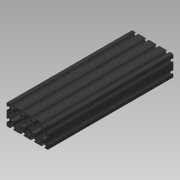
# Autodesk Inventor part: 2040
Saved by Autodesk Inventor 2013 (Build 170138000, 138)
## iProperties
Company: 80/20 Inc.
Created: 2013-09-06
Part Number: 2040
Material: Generic
Document SubType Name: Modeling
Density: 1 g/cm^3
Catalog Web Link: 8020.net
Vendor: 80/20 Inc.
Engineer: Ross Bowman
Author: Ross Bowman
Keywords: T-Slot, Extrusion, 80/20, 8020, Quick Frame, HT
Autodesk Inventor part; units mm, degrees
ref_plane "YZ Plane" through (0, 0, 0) normal (1, 0, 0) x (0, 1, 0)
ref_plane "XZ Plane" through (0, 0, 0) normal (0, 1, 0) x (-1, 0, 0)
ref_plane "XY Plane" through (0, 0, 0) normal (0, 0, 1) x (1, 0, 0)
sketch "Sketch1" plane through (0, 0, 0) normal (0, 0, 1) x (1, 0, 0)
  circle A0 centre (-12.7, 12.7) radius 2.6035
  circle A1 centre (-12.7, -12.7) radius 2.6035
  circle A2 centre (-38.1, 12.7) radius 2.6035
  circle A3 centre (-38.1, -12.7) radius 2.6035
  circle A4 centre (12.7, 12.7) radius 2.6035
  circle A5 centre (12.7, -12.7) radius 2.6035
  circle A6 centre (38.1, 12.7) radius 2.6035
  circle A7 centre (38.1, -12.7) radius 2.6035
  line L0 (-7.2742, 8.8373) -> (-2.0654, 3.6286)
  arc A8 (-2.0654, 3.6286) -> (2.0654, 3.6286) centre (0, 5.6941) ccw
  line L1 (2.0654, 3.6286) -> (7.2742, 8.8373)
  arc A9 (7.2742, 8.8373) -> (8.2042, 11.0824) centre (5.0292, 11.0824) ccw
  line L2 (8.2042, 11.0824) -> (8.2042, 14.3186)
  arc A10 (8.2042, 14.3186) -> (7.2743, 16.5636) centre (5.0292, 14.3186) ccw
  line L3 (7.2743, 16.5636) -> (2.0655, 21.7725)
  arc A11 (2.0655, 21.7725) -> (-2.0655, 21.7725) centre (0, 19.7071) ccw
  line L4 (-2.0655, 21.7725) -> (-7.2743, 16.5636)
  arc A12 (-7.2743, 16.5636) -> (-8.2042, 14.3186) centre (-5.0292, 14.3186) ccw
  line L5 (-8.2042, 14.3186) -> (-8.2042, 11.0824)
  arc A13 (-8.2042, 11.0824) -> (-7.2742, 8.8373) centre (-5.0292, 11.0824) ccw
  line L6 (-7.2743, -16.5636) -> (-2.0655, -21.7725)
  arc A14 (-2.0655, -21.7725) -> (2.0655, -21.7725) centre (0, -19.7071) ccw
  line L7 (2.0655, -21.7725) -> (7.2743, -16.5636)
  arc A15 (7.2743, -16.5636) -> (8.2042, -14.3186) centre (5.0292, -14.3186) ccw
  line L8 (8.2042, -14.3186) -> (8.2042, -11.0824)
  arc A16 (8.2042, -11.0824) -> (7.2742, -8.8373) centre (5.0292, -11.0824) ccw
  line L9 (7.2742, -8.8373) -> (2.0654, -3.6286)
  arc A17 (2.0654, -3.6286) -> (-2.0654, -3.6286) centre (0, -5.6941) ccw
  line L10 (-2.0654, -3.6286) -> (-7.2742, -8.8373)
  arc A18 (-7.2742, -8.8373) -> (-8.2042, -11.0824) centre (-5.0292, -11.0824) ccw
  line L11 (-8.2042, -11.0824) -> (-8.2042, -14.3186)
  arc A19 (-8.2042, -14.3186) -> (-7.2743, -16.5636) centre (-5.0292, -14.3186) ccw
  line L12 (-17.1958, 10.414) -> (-17.1958, 14.7184)
  arc A20 (-17.1958, 14.7184) -> (-17.843, 16.2809) centre (-19.4056, 14.7184) ccw
  line L13 (-17.843, 16.2809) -> (-23.3345, 21.7725)
  arc A21 (-23.3345, 21.7725) -> (-27.4655, 21.7725) centre (-25.4, 19.7071) ccw
  line L14 (-27.4655, 21.7725) -> (-32.957, 16.2809)
  arc A22 (-32.957, 16.2809) -> (-33.6042, 14.7184) centre (-31.3944, 14.7184) ccw
  line L15 (-33.6042, 14.7184) -> (-33.6042, 10.414)
  arc A23 (-35.814, 8.2042) -> (-33.6042, 10.414) centre (-35.814, 10.414) ccw
  line L16 (-35.814, 8.2042) -> (-40.1184, 8.2042)
  arc A24 (-40.1184, 8.2042) -> (-41.6809, 7.557) centre (-40.1184, 5.9944) ccw
  line L17 (-41.6809, 7.557) -> (-47.1725, 2.0655)
  arc A25 (-47.1725, 2.0655) -> (-47.1725, -2.0655) centre (-45.1071, 0) ccw
  line L18 (-47.1725, -2.0655) -> (-41.6809, -7.557)
  arc A26 (-41.6809, -7.557) -> (-40.1184, -8.2042) centre (-40.1184, -5.9944) ccw
  line L19 (-40.1184, -8.2042) -> (-35.814, -8.2042)
  arc A27 (-33.6042, -10.414) -> (-35.814, -8.2042) centre (-35.814, -10.414) ccw
  line L20 (-33.6042, -10.414) -> (-33.6042, -14.7184)
  arc A28 (-33.6042, -14.7184) -> (-32.957, -16.2809) centre (-31.3944, -14.7184) ccw
  line L21 (-32.957, -16.2809) -> (-27.4655, -21.7725)
  arc A29 (-27.4655, -21.7725) -> (-23.3345, -21.7725) centre (-25.4, -19.7071) ccw
  line L22 (-23.3345, -21.7725) -> (-17.843, -16.2809)
  arc A30 (-17.843, -16.2809) -> (-17.1958, -14.7184) centre (-19.4056, -14.7184) ccw
  line L23 (-17.1958, -14.7184) -> (-17.1958, -10.414)
  arc A31 (-14.986, -8.2042) -> (-17.1958, -10.414) centre (-14.986, -10.414) ccw
  line L24 (-14.986, -8.2042) -> (-10.6816, -8.2042)
  arc A32 (-10.6816, -8.2042) -> (-9.1191, -7.557) centre (-10.6816, -5.9944) ccw
  line L25 (-9.1191, -7.557) -> (-3.6275, -2.0655)
  arc A33 (-3.6275, -2.0655) -> (-3.6275, 2.0655) centre (-5.6929, 0) ccw
  line L26 (-3.6275, 2.0655) -> (-9.1191, 7.557)
  arc A34 (-9.1191, 7.557) -> (-10.6816, 8.2042) centre (-10.6816, 5.9944) ccw
  line L27 (-10.6816, 8.2042) -> (-14.986, 8.2042)
  arc A35 (-17.1958, 10.414) -> (-14.986, 8.2042) centre (-14.986, 10.414) ccw
  line L28 (14.986, 8.2042) -> (10.6816, 8.2042)
  arc A36 (10.6816, 8.2042) -> (9.1191, 7.557) centre (10.6816, 5.9944) ccw
  line L29 (9.1191, 7.557) -> (3.6275, 2.0655)
  arc A37 (3.6275, 2.0655) -> (3.6275, -2.0655) centre (5.6929, 0) ccw
  line L30 (3.6275, -2.0655) -> (9.1191, -7.557)
  arc A38 (9.1191, -7.557) -> (10.6816, -8.2042) centre (10.6816, -5.9944) ccw
  line L31 (10.6816, -8.2042) -> (14.986, -8.2042)
  arc A39 (17.1958, -10.414) -> (14.986, -8.2042) centre (14.986, -10.414) ccw
  line L32 (17.1958, -10.414) -> (17.1958, -14.7184)
  arc A40 (17.1958, -14.7184) -> (17.843, -16.2809) centre (19.4056, -14.7184) ccw
  line L33 (17.843, -16.2809) -> (23.3345, -21.7725)
  arc A41 (23.3345, -21.7725) -> (27.4655, -21.7725) centre (25.4, -19.7071) ccw
  line L34 (27.4655, -21.7725) -> (32.957, -16.2809)
  line L35 (33.6042, -14.7184) -> (33.6042, -10.414)
  arc A42 (35.814, -8.2042) -> (33.6042, -10.414) centre (35.814, -10.414) ccw
  line L36 (35.814, -8.2042) -> (40.1184, -8.2042)
  arc A43 (40.1184, -8.2042) -> (41.6809, -7.557) centre (40.1184, -5.9944) ccw
  line L37 (41.6809, -7.557) -> (47.1725, -2.0655)
  arc A44 (47.1725, -2.0655) -> (47.1725, 2.0655) centre (45.1071, 0) ccw
  line L38 (47.1725, 2.0655) -> (41.6809, 7.557)
  arc A45 (41.6809, 7.557) -> (40.1184, 8.2042) centre (40.1184, 5.9944) ccw
  line L39 (40.1184, 8.2042) -> (35.814, 8.2042)
  arc A46 (33.6042, 10.414) -> (35.814, 8.2042) centre (35.814, 10.414) ccw
  line L40 (33.6042, 10.414) -> (33.6042, 14.7184)
  arc A47 (33.6042, 14.7184) -> (32.957, 16.2809) centre (31.3944, 14.7184) ccw
  line L41 (32.957, 16.2809) -> (27.4655, 21.7725)
  arc A48 (27.4655, 21.7725) -> (23.3345, 21.7725) centre (25.4, 19.7071) ccw
  line L42 (23.3345, 21.7725) -> (17.843, 16.2809)
  arc A49 (17.843, 16.2809) -> (17.1958, 14.7184) centre (19.4056, 14.7184) ccw
  line L43 (17.1958, 14.7184) -> (17.1958, 10.414)
  arc A50 (14.986, 8.2042) -> (17.1958, 10.414) centre (14.986, 10.414) ccw
  arc A51 (32.957, -16.2809) -> (33.6042, -14.7184) centre (31.3944, -14.7184) ccw
  line L44 (2.1336, 25.4) -> (-2.1336, 25.4)
  arc A52 (-3.1496, 25.4) -> (-2.1336, 25.4) centre (-2.6416, 25.4) ccw
  line L45 (-3.1496, 25.4) -> (-6.096, 25.4)
  arc A53 (-7.112, 25.4) -> (-6.096, 25.4) centre (-6.604, 25.4) ccw
  line L46 (-7.112, 25.4) -> (-8.3566, 25.4)
  arc A54 (-8.3566, 25.4) -> (-8.3566, 23.1902) centre (-8.357, 24.2951) ccw
  line L47 (-8.3566, 23.1902) -> (-6.2257, 23.1902)
  arc A55 (-5.5073, 21.4558) -> (-6.2257, 23.1902) centre (-6.2257, 22.1742) ccw
  line L48 (-5.5073, 21.4558) -> (-8.8373, 18.1258)
  arc A56 (-11.0824, 17.1958) -> (-8.8373, 18.1258) centre (-11.0824, 20.3708) ccw
  line L49 (-11.0824, 17.1958) -> (-14.3176, 17.1958)
  arc A57 (-16.5627, 18.1258) -> (-14.3176, 17.1958) centre (-14.3176, 20.3708) ccw
  line L50 (-16.5627, 18.1258) -> (-19.8927, 21.4558)
  arc A58 (-19.1743, 23.1902) -> (-19.8927, 21.4558) centre (-19.1743, 22.1742) ccw
  line L51 (-19.1743, 23.1902) -> (-17.0434, 23.1902)
  arc A59 (-17.0434, 23.1902) -> (-17.0434, 25.4) centre (-17.0441, 24.2951) ccw
  line L52 (-17.0434, 25.4) -> (-18.288, 25.4)
  arc A60 (-19.304, 25.4) -> (-18.288, 25.4) centre (-18.796, 25.4) ccw
  line L53 (-19.304, 25.4) -> (-22.2504, 25.4)
  arc A61 (-23.2664, 25.4) -> (-22.2504, 25.4) centre (-22.7584, 25.4) ccw
  line L54 (-23.2664, 25.4) -> (-27.5336, 25.4)
  arc A62 (-28.5496, 25.4) -> (-27.5336, 25.4) centre (-28.0416, 25.4) ccw
  line L55 (-28.5496, 25.4) -> (-31.496, 25.4)
  arc A63 (-32.512, 25.4) -> (-31.496, 25.4) centre (-32.004, 25.4) ccw
  line L56 (-32.512, 25.4) -> (-33.7566, 25.4)
  arc A64 (-33.7566, 25.4) -> (-33.7566, 23.1902) centre (-33.757, 24.2951) ccw
  line L57 (-33.7566, 23.1902) -> (-31.6257, 23.1902)
  arc A65 (-30.9073, 21.4558) -> (-31.6257, 23.1902) centre (-31.6257, 22.1742) ccw
  line L58 (-30.9073, 21.4558) -> (-34.2373, 18.1258)
  arc A66 (-36.4824, 17.1958) -> (-34.2373, 18.1258) centre (-36.4824, 20.3708) ccw
  line L59 (-36.4824, 17.1958) -> (-39.7176, 17.1958)
  arc A67 (-41.9627, 18.1258) -> (-39.7176, 17.1958) centre (-39.7176, 20.3708) ccw
  line L60 (-41.9627, 18.1258) -> (-45.2927, 21.4558)
  arc A68 (-44.5743, 23.1902) -> (-45.2927, 21.4558) centre (-44.5743, 22.1742) ccw
  line L61 (-44.5743, 23.1902) -> (-42.4434, 23.1902)
  arc A69 (-42.4434, 23.1902) -> (-42.4434, 25.4) centre (-42.4441, 24.2951) ccw
  line L62 (-42.4434, 25.4) -> (-43.688, 25.4)
  arc A70 (-44.704, 25.4) -> (-43.688, 25.4) centre (-44.196, 25.4) ccw
  line L63 (-44.704, 25.4) -> (-47.6504, 25.4)
  arc A71 (-48.6664, 25.3998) -> (-47.6504, 25.4) centre (-48.1584, 25.4001) ccw
  arc A72 (-48.6664, 25.3998) -> (-50.8011, 23.2664) centre (-48.6931, 23.2918) ccw
  arc A73 (-50.8, 22.2504) -> (-50.8011, 23.2664) centre (-50.8, 22.7584) ccw
  line L64 (-50.8, 22.2504) -> (-50.8, 19.304)
  arc A74 (-50.8, 18.288) -> (-50.8, 19.304) centre (-50.8, 18.796) ccw
  line L65 (-50.8, 18.288) -> (-50.8, 17.0434)
  arc A75 (-50.8, 17.0434) -> (-48.5902, 17.0434) centre (-49.6951, 17.0438) ccw
  line L66 (-48.5902, 17.0434) -> (-48.5902, 19.1743)
  arc A76 (-46.8558, 19.8927) -> (-48.5902, 19.1743) centre (-47.5742, 19.1743) ccw
  line L67 (-46.8558, 19.8927) -> (-43.5258, 16.5627)
  arc A77 (-42.5958, 14.3176) -> (-43.5258, 16.5627) centre (-45.7708, 14.3176) ccw
  line L68 (-42.5958, 14.3176) -> (-42.5958, 11.0824)
  arc A78 (-43.5258, 8.8373) -> (-42.5958, 11.0824) centre (-45.7708, 11.0824) ccw
  line L69 (-43.5258, 8.8373) -> (-46.8558, 5.5073)
  arc A79 (-48.5902, 6.2257) -> (-46.8558, 5.5073) centre (-47.5742, 6.2257) ccw
  line L70 (-48.5902, 6.2257) -> (-48.5902, 8.3566)
  arc A80 (-48.5902, 8.3566) -> (-50.8, 8.3566) centre (-49.6951, 8.3573) ccw
  line L71 (-50.8, 8.3566) -> (-50.8, 7.112)
  arc A81 (-50.8, 6.096) -> (-50.8, 7.112) centre (-50.8, 6.604) ccw
  line L72 (-50.8, 6.096) -> (-50.8, 3.1496)
  arc A82 (-50.8, 2.1336) -> (-50.8, 3.1496) centre (-50.8, 2.6416) ccw
  line L73 (-50.8, 2.1336) -> (-50.8, -2.1336)
  arc A83 (-50.8, -3.1496) -> (-50.8, -2.1336) centre (-50.8, -2.6416) ccw
  line L74 (-50.8, -3.1496) -> (-50.8, -6.096)
  arc A84 (-50.8, -7.112) -> (-50.8, -6.096) centre (-50.8, -6.604) ccw
  line L75 (-50.8, -7.112) -> (-50.8, -8.3566)
  arc A85 (-50.8, -8.3566) -> (-48.5902, -8.3566) centre (-49.6951, -8.3562) ccw
  line L76 (-48.5902, -8.3566) -> (-48.5902, -6.2257)
  arc A86 (-46.8558, -5.5073) -> (-48.5902, -6.2257) centre (-47.5742, -6.2257) ccw
  line L77 (-46.8558, -5.5073) -> (-43.5258, -8.8373)
  arc A87 (-42.5958, -11.0824) -> (-43.5258, -8.8373) centre (-45.7708, -11.0824) ccw
  line L78 (-42.5958, -11.0824) -> (-42.5958, -14.3176)
  arc A88 (-43.5258, -16.5627) -> (-42.5958, -14.3176) centre (-45.7708, -14.3176) ccw
  line L79 (-43.5258, -16.5627) -> (-46.8558, -19.8927)
  arc A89 (-48.5902, -19.1743) -> (-46.8558, -19.8927) centre (-47.5742, -19.1743) ccw
  line L80 (-48.5902, -19.1743) -> (-48.5902, -17.0434)
  arc A90 (-48.5902, -17.0434) -> (-50.8, -17.0434) centre (-49.6951, -17.0427) ccw
  line L81 (-50.8, -17.0434) -> (-50.8, -18.288)
  arc A91 (-50.8, -19.304) -> (-50.8, -18.288) centre (-50.8, -18.796) ccw
  line L82 (-50.8, -19.304) -> (-50.8, -22.2504)
  arc A92 (-50.7998, -23.2664) -> (-50.8, -22.2504) centre (-50.8, -22.7584) ccw
  arc A93 (-50.7998, -23.2664) -> (-48.6664, -25.3998) centre (-48.6918, -23.2918) ccw
  arc A94 (-47.6504, -25.4) -> (-48.6664, -25.3998) centre (-48.1584, -25.4) ccw
  line L83 (-47.6504, -25.4) -> (-44.704, -25.4)
  arc A95 (-43.688, -25.4) -> (-44.704, -25.4) centre (-44.196, -25.4) ccw
  line L84 (-43.688, -25.4) -> (-42.4434, -25.4)
  arc A96 (-42.4434, -25.4) -> (-42.4434, -23.1902) centre (-42.4441, -24.2951) ccw
  line L85 (-42.4434, -23.1902) -> (-44.5743, -23.1902)
  arc A97 (-45.2927, -21.4558) -> (-44.5743, -23.1902) centre (-44.5743, -22.1742) ccw
  line L86 (-45.2927, -21.4558) -> (-41.9627, -18.1258)
  arc A98 (-39.7176, -17.1958) -> (-41.9627, -18.1258) centre (-39.7176, -20.3708) ccw
  line L87 (-39.7176, -17.1958) -> (-36.4824, -17.1958)
  arc A99 (-34.2373, -18.1258) -> (-36.4824, -17.1958) centre (-36.4824, -20.3708) ccw
  line L88 (-34.2373, -18.1258) -> (-30.9073, -21.4558)
  arc A100 (-31.6257, -23.1902) -> (-30.9073, -21.4558) centre (-31.6257, -22.1742) ccw
  line L89 (-31.6257, -23.1902) -> (-33.7566, -23.1902)
  arc A101 (-33.7566, -23.1902) -> (-33.7566, -25.4) centre (-33.7575, -24.2951) ccw
  line L90 (-33.7566, -25.4) -> (-32.512, -25.4)
  arc A102 (-31.496, -25.4) -> (-32.512, -25.4) centre (-32.004, -25.4) ccw
  line L91 (-31.496, -25.4) -> (-28.5496, -25.4)
  arc A103 (-27.5336, -25.4) -> (-28.5496, -25.4) centre (-28.0416, -25.4) ccw
  line L92 (-27.5336, -25.4) -> (-23.2664, -25.4)
  arc A104 (-22.2504, -25.4) -> (-23.2664, -25.4) centre (-22.7584, -25.4) ccw
  line L93 (-22.2504, -25.4) -> (-19.304, -25.4)
  arc A105 (-18.288, -25.4) -> (-19.304, -25.4) centre (-18.796, -25.4) ccw
  line L94 (-18.288, -25.4) -> (-17.0434, -25.4)
  arc A106 (-17.0434, -25.4) -> (-17.0434, -23.1902) centre (-17.0441, -24.2951) ccw
  line L95 (-17.0434, -23.1902) -> (-19.1743, -23.1902)
  arc A107 (-19.8927, -21.4558) -> (-19.1743, -23.1902) centre (-19.1743, -22.1742) ccw
  line L96 (-19.8927, -21.4558) -> (-16.5627, -18.1258)
  arc A108 (-14.3176, -17.1958) -> (-16.5627, -18.1258) centre (-14.3176, -20.3708) ccw
  line L97 (-14.3176, -17.1958) -> (-11.0824, -17.1958)
  arc A109 (-8.8373, -18.1258) -> (-11.0824, -17.1958) centre (-11.0824, -20.3708) ccw
  line L98 (-8.8373, -18.1258) -> (-5.5073, -21.4558)
  arc A110 (-6.2257, -23.1902) -> (-5.5073, -21.4558) centre (-6.2257, -22.1742) ccw
  line L99 (-6.2257, -23.1902) -> (-8.3566, -23.1902)
  arc A111 (-8.3566, -23.1902) -> (-8.3566, -25.4) centre (-8.3575, -24.2951) ccw
  line L100 (-8.3566, -25.4) -> (-7.112, -25.4)
  arc A112 (-6.096, -25.4) -> (-7.112, -25.4) centre (-6.604, -25.4) ccw
  line L101 (-6.096, -25.4) -> (-3.1496, -25.4)
  arc A113 (-2.1336, -25.4) -> (-3.1496, -25.4) centre (-2.6416, -25.4) ccw
  line L102 (-2.1336, -25.4) -> (2.1336, -25.4)
  arc A114 (3.1496, -25.4) -> (2.1336, -25.4) centre (2.6416, -25.4) ccw
  line L103 (3.1496, -25.4) -> (6.096, -25.4)
  arc A115 (7.112, -25.4) -> (6.096, -25.4) centre (6.604, -25.4) ccw
  line L104 (7.112, -25.4) -> (8.3566, -25.4)
  arc A116 (8.3566, -25.4) -> (8.3566, -23.1902) centre (8.3559, -24.2951) ccw
  line L105 (8.3566, -23.1902) -> (6.2257, -23.1902)
  arc A117 (5.5073, -21.4558) -> (6.2257, -23.1902) centre (6.2257, -22.1742) ccw
  line L106 (5.5073, -21.4558) -> (8.8373, -18.1258)
  arc A118 (11.0824, -17.1958) -> (8.8373, -18.1258) centre (11.0824, -20.3708) ccw
  line L107 (11.0824, -17.1958) -> (14.3176, -17.1958)
  arc A119 (16.5627, -18.1258) -> (14.3176, -17.1958) centre (14.3176, -20.3708) ccw
  line L108 (16.5627, -18.1258) -> (19.8927, -21.4558)
  arc A120 (19.1743, -23.1902) -> (19.8927, -21.4558) centre (19.1743, -22.1742) ccw
  line L109 (19.1743, -23.1902) -> (17.0434, -23.1902)
  arc A121 (17.0434, -23.1902) -> (17.0434, -25.4) centre (17.0425, -24.2951) ccw
  line L110 (17.0434, -25.4) -> (18.288, -25.4)
  arc A122 (19.304, -25.4) -> (18.288, -25.4) centre (18.796, -25.4) ccw
  line L111 (19.304, -25.4) -> (22.2504, -25.4)
  arc A123 (23.2664, -25.4) -> (22.2504, -25.4) centre (22.7584, -25.4) ccw
  line L112 (23.2664, -25.4) -> (27.5336, -25.4)
  arc A124 (28.5496, -25.4) -> (27.5336, -25.4) centre (28.0416, -25.4) ccw
  line L113 (28.5496, -25.4) -> (31.496, -25.4)
  arc A125 (32.512, -25.4) -> (31.496, -25.4) centre (32.004, -25.4) ccw
  line L114 (32.512, -25.4) -> (33.7566, -25.4)
  arc A126 (33.7566, -25.4) -> (33.7566, -23.1902) centre (33.7559, -24.2951) ccw
  line L115 (33.7566, -23.1902) -> (31.6257, -23.1902)
  arc A127 (30.9073, -21.4558) -> (31.6257, -23.1902) centre (31.6257, -22.1742) ccw
  line L116 (30.9073, -21.4558) -> (34.2373, -18.1258)
  arc A128 (36.4824, -17.1958) -> (34.2373, -18.1258) centre (36.4824, -20.3708) ccw
  line L117 (36.4824, -17.1958) -> (39.7176, -17.1958)
  arc A129 (41.9627, -18.1258) -> (39.7176, -17.1958) centre (39.7176, -20.3708) ccw
  line L118 (41.9627, -18.1258) -> (45.2927, -21.4558)
  arc A130 (44.5743, -23.1902) -> (45.2927, -21.4558) centre (44.5743, -22.1742) ccw
  line L119 (44.5743, -23.1902) -> (42.4434, -23.1902)
  arc A131 (42.4434, -23.1902) -> (42.4434, -25.4) centre (42.4425, -24.2951) ccw
  line L120 (42.4434, -25.4) -> (43.688, -25.4)
  arc A132 (44.704, -25.4) -> (43.688, -25.4) centre (44.196, -25.4) ccw
  line L121 (44.704, -25.4) -> (47.6504, -25.4)
  arc A133 (48.6664, -25.3998) -> (47.6504, -25.4) centre (48.1584, -25.4) ccw
  arc A134 (48.6664, -25.3998) -> (50.7998, -23.2664) centre (48.6918, -23.2918) ccw
  arc A135 (50.8, -22.2504) -> (50.7998, -23.2664) centre (50.8, -22.7584) ccw
  line L122 (50.8, -22.2504) -> (50.8, -19.304)
  arc A136 (50.8, -18.288) -> (50.8, -19.304) centre (50.8, -18.796) ccw
  line L123 (50.8, -18.288) -> (50.8, -17.0434)
  arc A137 (50.8, -17.0434) -> (48.5902, -17.0434) centre (49.6951, -17.043) ccw
  line L124 (48.5902, -17.0434) -> (48.5902, -19.1743)
  arc A138 (46.8558, -19.8927) -> (48.5902, -19.1743) centre (47.5742, -19.1742) ccw
  line L125 (46.8558, -19.8927) -> (43.5258, -16.5627)
  arc A139 (42.5958, -14.3176) -> (43.5258, -16.5627) centre (45.7708, -14.3176) ccw
  line L126 (42.5958, -14.3176) -> (42.5958, -11.0824)
  arc A140 (43.5258, -8.8373) -> (42.5958, -11.0824) centre (45.7708, -11.0824) ccw
  line L127 (43.5258, -8.8373) -> (46.8558, -5.5073)
  arc A141 (48.5902, -6.2257) -> (46.8558, -5.5073) centre (47.5742, -6.2257) ccw
  line L128 (48.5902, -6.2257) -> (48.5902, -8.3566)
  arc A142 (48.5902, -8.3566) -> (50.8, -8.3566) centre (49.6951, -8.355) ccw
  line L129 (50.8, -8.3566) -> (50.8, -7.112)
  arc A143 (50.8, -6.096) -> (50.8, -7.112) centre (50.8, -6.604) ccw
  line L130 (50.8, -6.096) -> (50.8, -3.1496)
  arc A144 (50.8, -2.1336) -> (50.8, -3.1496) centre (50.8, -2.6416) ccw
  line L131 (50.8, -2.1336) -> (50.8, 2.1336)
  arc A145 (50.8, 3.1496) -> (50.8, 2.1336) centre (50.8, 2.6416) ccw
  line L132 (50.8, 3.1496) -> (50.8, 6.096)
  arc A146 (50.8, 7.112) -> (50.8, 6.096) centre (50.8, 6.604) ccw
  line L133 (50.8, 7.112) -> (50.8, 8.3566)
  arc A147 (50.8, 8.3566) -> (48.5902, 8.3566) centre (49.6951, 8.357) ccw
  line L134 (48.5902, 8.3566) -> (48.5902, 6.2258)
  arc A148 (46.8558, 5.5073) -> (48.5902, 6.2258) centre (47.5742, 6.2258) ccw
  line L135 (46.8558, 5.5073) -> (43.5258, 8.8373)
  arc A149 (42.5958, 11.0824) -> (43.5258, 8.8373) centre (45.7708, 11.0824) ccw
  line L136 (42.5958, 11.0824) -> (42.5958, 14.3176)
  arc A150 (43.5258, 16.5627) -> (42.5958, 14.3176) centre (45.7708, 14.3176) ccw
  line L137 (43.5258, 16.5627) -> (46.8558, 19.8927)
  arc A151 (48.5902, 19.1743) -> (46.8558, 19.8927) centre (47.5742, 19.1743) ccw
  line L138 (48.5902, 19.1743) -> (48.5902, 17.0434)
  arc A152 (48.5902, 17.0434) -> (50.8, 17.0434) centre (49.6951, 17.045) ccw
  line L139 (50.8, 17.0434) -> (50.8, 18.288)
  arc A153 (50.8, 19.304) -> (50.8, 18.288) centre (50.8, 18.796) ccw
  line L140 (50.8, 19.304) -> (50.8, 22.2504)
  arc A154 (50.7998, 23.2664) -> (50.8, 22.2504) centre (50.8001, 22.7584) ccw
  arc A155 (50.7998, 23.2664) -> (48.6664, 25.3999) centre (48.6918, 23.2918) ccw
  arc A156 (47.6504, 25.4) -> (48.6664, 25.3999) centre (48.1584, 25.4) ccw
  line L141 (47.6504, 25.4) -> (44.704, 25.4)
  arc A157 (43.688, 25.4) -> (44.704, 25.4) centre (44.196, 25.4) ccw
  line L142 (43.688, 25.4) -> (42.4434, 25.4)
  arc A158 (42.4434, 25.4) -> (42.4434, 23.1902) centre (42.443, 24.2951) ccw
  line L143 (42.4434, 23.1902) -> (44.5743, 23.1902)
  arc A159 (45.2927, 21.4558) -> (44.5743, 23.1902) centre (44.5743, 22.1742) ccw
  line L144 (45.2927, 21.4558) -> (41.9627, 18.1258)
  arc A160 (39.7176, 17.1958) -> (41.9627, 18.1258) centre (39.7176, 20.3708) ccw
  line L145 (39.7176, 17.1958) -> (36.4824, 17.1958)
  arc A161 (34.2373, 18.1258) -> (36.4824, 17.1958) centre (36.4824, 20.3708) ccw
  line L146 (34.2373, 18.1258) -> (30.9073, 21.4558)
  arc A162 (31.6257, 23.1902) -> (30.9073, 21.4558) centre (31.6257, 22.1742) ccw
  line L147 (31.6257, 23.1902) -> (33.7566, 23.1902)
  arc A163 (33.7566, 23.1902) -> (33.7566, 25.4) centre (33.7559, 24.2951) ccw
  line L148 (33.7566, 25.4) -> (32.512, 25.4)
  arc A164 (31.496, 25.4) -> (32.512, 25.4) centre (32.004, 25.4) ccw
  line L149 (31.496, 25.4) -> (28.5496, 25.4)
  arc A165 (27.5336, 25.4) -> (28.5496, 25.4) centre (28.0416, 25.4) ccw
  line L150 (27.5336, 25.4) -> (23.2664, 25.4)
  arc A166 (22.2504, 25.4) -> (23.2664, 25.4) centre (22.7584, 25.4) ccw
  line L151 (22.2504, 25.4) -> (19.304, 25.4)
  arc A167 (18.288, 25.4) -> (19.304, 25.4) centre (18.796, 25.4) ccw
  line L152 (18.288, 25.4) -> (17.0434, 25.4)
  arc A168 (17.0434, 25.4) -> (17.0434, 23.1902) centre (17.043, 24.2951) ccw
  line L153 (17.0434, 23.1902) -> (19.1743, 23.1902)
  arc A169 (19.8927, 21.4558) -> (19.1743, 23.1902) centre (19.1743, 22.1742) ccw
  line L154 (19.8927, 21.4558) -> (16.5627, 18.1258)
  arc A170 (14.3176, 17.1958) -> (16.5627, 18.1258) centre (14.3176, 20.3708) ccw
  line L155 (14.3176, 17.1958) -> (11.0824, 17.1958)
  arc A171 (8.8373, 18.1258) -> (11.0824, 17.1958) centre (11.0824, 20.3708) ccw
  line L156 (8.8373, 18.1258) -> (5.5073, 21.4558)
  arc A172 (6.2257, 23.1902) -> (5.5073, 21.4558) centre (6.2257, 22.1742) ccw
  line L157 (6.2257, 23.1902) -> (8.3566, 23.1902)
  arc A173 (8.3566, 23.1902) -> (8.3566, 25.4) centre (8.3559, 24.2951) ccw
  line L158 (8.3566, 25.4) -> (7.112, 25.4)
  arc A174 (6.096, 25.4) -> (7.112, 25.4) centre (6.604, 25.4) ccw
  line L159 (6.096, 25.4) -> (3.1496, 25.4)
  arc A175 (2.1336, 25.4) -> (3.1496, 25.4) centre (2.6416, 25.4007) ccw
  point P0 (0, 0)
  constraints: 336 point on circle, 320 end point, 176 centre point
extrude "Extrusion1" add sketch "Sketch1" against normal blind 304.8
body "Solid1"
